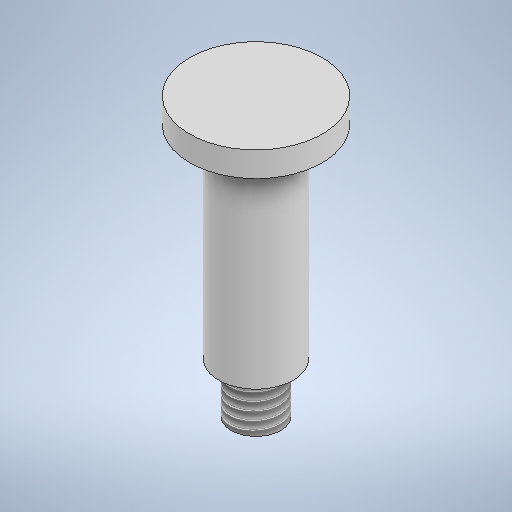
# Autodesk Inventor part: 2025
Saved by Autodesk Inventor 2025.1 (Build 291241000, 241)
## iProperties
Created: 2024-05-30
Part Number: 2025
Material: Generic
Document SubType Name: Modeling
Designer: Fabri
Density: 1 g/cm^3
Appearance: Default
Author: Fabri
Autodesk Inventor part; units mm, degrees
ref_plane "YZ Plane" through (0, 0, 0) normal (1, 0, 0) x (0, 1, 0)
ref_plane "XZ Plane" through (0, 0, 0) normal (0, 1, 0) x (-1, 0, 0)
ref_plane "XY Plane" through (0, 0, 0) normal (0, 0, 1) x (1, 0, 0)
sketch "Sketch1" plane through (0, 0, 0) normal (0, 1, 0) x (-1, 0, 0)
  line L0 (0, 0) -> (8, 0)
  line L1 (8, 0) -> (8, -3)
  line L2 (8, -3) -> (4.5, -3)
  line L3 (4.5, -3) -> (4.5, -27.5)
  line L4 (4.5, -27.5) -> (3, -27.5)
  line L5 (3, -27.5) -> (3, -33.5)
  line L6 (3, -33.5) -> (0, -33.5)
  line L7 (0, -33.5) -> (0, 0)
  point P0 (0, -16.75)
  dimension "d0" = 6
  dimension "d1" = 6
  dimension "d2" = 24.5
  dimension "d3" = 3
  dimension "d4" = 9
  dimension "d5" = 16
  constraints: 16 end point, 7 perpendicular, 1 horizontal, 1 midpoint
  measures "d0" diameter of L5 L7
  measures "d1" distance between parallel lines of L6 L4
  measures "d2" distance of L2.end L3.end
  measures "d3" distance of L0.end L1.end
  measures "d4" diameter of L3 point (0, -16.75)
  measures "d5" diameter of L1 L7
revolve "Revolution1" add sketch "Sketch1" angle 360 about axis through (0, 0, -33.5) along (0, 0, 1)
thread "Thread1" size "M6x1" class "6g" standard "ISO Metric profile" length 12
body "Solid1"
